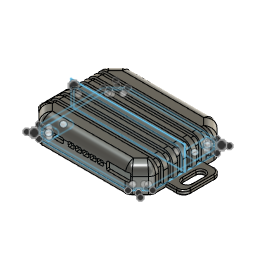
stm32-sensorleap-box-v12 (Autodesk Fusion 360 design; units mm, degrees)
Autodesk Fusion 360 part; units mm, degrees
sketch "Sketch1" plane through (0, 0, 0) normal (0, 0, 1) x (1, 0, 0) in component "lid"
  line L0 (-17.6716, 17.5) -> (17.6716, 17.5)
  line L1 (22, 13.1716) -> (22, -13.1716)
  line L2 (17.6716, -17.5) -> (-17.6716, -17.5)
  line L3 (-22, -13.1716) -> (-22, 13.1716)
  line L4 (-17.5574, 18.8) -> (17.5574, 18.8)
  line L5 (24, 12.3574) -> (24, -12.3074)
  line L6 (17.5574, -18.75) -> (-17.5574, -18.75)
  line L7 (-24, -12.3074) -> (-24, 12.3574)
  line L8 (19.0858, 16.9142) -> (21.4142, 14.5858)
  line L9 (21.4142, -14.5858) -> (19.0858, -16.9142)
  line L10 (-19.0858, -16.9142) -> (-21.4142, -14.5858)
  line L11 (-19.0858, 16.9142) -> (-21.4142, 14.5858)
  line L12 (19.6787, 17.9213) -> (23.1213, 14.4787)
  line L13 (23.1213, -14.4287) -> (19.6787, -17.8713)
  line L14 (-19.6787, -17.8713) -> (-23.1213, -14.4287)
  line L15 (-19.6787, 17.9213) -> (-23.1213, 14.4787)
  arc A0 (19.0858, 16.9142) -> (17.6716, 17.5) centre (17.6716, 15.5) ccw
  arc A1 (22, 13.1716) -> (21.4142, 14.5858) centre (20, 13.1716) ccw
  arc A2 (21.4142, -14.5858) -> (22, -13.1716) centre (20, -13.1716) ccw
  arc A3 (17.6716, -17.5) -> (19.0858, -16.9142) centre (17.6716, -15.5) ccw
  arc A4 (-19.0858, -16.9142) -> (-17.6716, -17.5) centre (-17.6716, -15.5) ccw
  arc A5 (-22, -13.1716) -> (-21.4142, -14.5858) centre (-20, -13.1716) ccw
  arc A6 (-21.4142, 14.5858) -> (-22, 13.1716) centre (-20, 13.1716) ccw
  arc A7 (-17.6716, 17.5) -> (-19.0858, 16.9142) centre (-17.6716, 15.5) ccw
  arc A8 (19.6787, 17.9213) -> (17.5574, 18.8) centre (17.5574, 15.8) ccw
  arc A9 (24, 12.3574) -> (23.1213, 14.4787) centre (21, 12.3574) ccw
  arc A10 (23.1213, -14.4287) -> (24, -12.3074) centre (21, -12.3074) ccw
  arc A11 (17.5574, -18.75) -> (19.6787, -17.8713) centre (17.5574, -15.75) ccw
  arc A12 (-19.6787, -17.8713) -> (-17.5574, -18.75) centre (-17.5574, -15.75) ccw
  arc A13 (-24, -12.3074) -> (-23.1213, -14.4287) centre (-21, -12.3074) ccw
  arc A14 (-23.1213, 14.4787) -> (-24, 12.3574) centre (-21, 12.3574) ccw
  arc A15 (-17.5574, 18.8) -> (-19.6787, 17.9213) centre (-17.5574, 15.8) ccw
  point P0 (-22, 17.5)
  point P1 (22, 17.5)
  point P2 (22, -17.5)
  point P3 (-22, -17.5)
  point P4 (-24, 18.8)
  point P5 (24, 18.8)
  point P6 (24, -18.75)
  point P7 (-24, -18.75)
  point P8 (18.5, 17.5)
  point P9 (22, 14)
  point P10 (22, -14)
  point P11 (18.5, -17.5)
  point P12 (-18.5, -17.5)
  point P13 (-22, -14)
  point P14 (-18.5, 17.5)
  point P15 (-22, 14)
  point P16 (18.8, 18.8)
  point P17 (24, 13.6)
  point P18 (24, -13.55)
  point P19 (18.8, -18.75)
  point P20 (-18.8, -18.75)
  point P21 (-24, -13.55)
  point P22 (-18.8, 18.8)
  point P23 (-24, 13.6)
  dimension "d1" = 44
  dimension "d2" = 35
  dimension "d3" = 3.5
  dimension "d4" = 3.5
  dimension "d5" = 3.5
  dimension "d6" = 3.5
  dimension "d7" = 3.5
  dimension "d8" = 3.5
  dimension "d9" = 3.5
  dimension "d10" = 3.5
  dimension "d11" = 5.2
  dimension "d12" = 5.2
  dimension "d13" = 5.2
  dimension "d14" = 5.2
  dimension "d15" = 5.2
  dimension "d16" = 5.2
  dimension "d17" = 5.2
  dimension "d18" = 5.2
  dimension "d19" = 2
  dimension "d20" = 3
  constraint horizontal L0
  constraint vertical L1
  constraint horizontal L2
  constraint vertical L3
  constraint horizontal L4
  constraint vertical L5
  constraint horizontal L6
  constraint vertical L7
  constraint coincident P1 L0
  constraint coincident P1 L1
  constraint coincident P2 L1
  constraint coincident P2 L2
  constraint coincident P3 L2
  constraint coincident P3 L3
  constraint coincident P0 L0
  constraint coincident P0 L3
  constraint coincident P5 L4
  constraint coincident P5 L5
  constraint coincident P6 L5
  constraint coincident P6 L6
  constraint coincident P7 L6
  constraint coincident P7 L7
  constraint coincident P4 L4
  constraint coincident P4 L7
  constraint coincident L0 P8
  constraint coincident P8 L8
  constraint tangent L0 A0
  constraint tangent L8 A0
  constraint coincident P9 L8
  constraint coincident L1 P9
  constraint tangent L8 A1
  constraint tangent L1 A1
  constraint equal A0 A1
  constraint coincident L1 P10
  constraint coincident P10 L9
  constraint tangent L1 A2
  constraint tangent L9 A2
  constraint equal A0 A2
  constraint coincident P11 L9
  constraint coincident L2 P11
  constraint tangent L9 A3
  constraint tangent L2 A3
  constraint equal A0 A3
  constraint coincident L2 P12
  constraint coincident P12 L10
  constraint tangent L2 A4
  constraint tangent L10 A4
  constraint equal A0 A4
  constraint coincident P13 L10
  constraint coincident L3 P13
  constraint tangent L10 A5
  constraint tangent L3 A5
  constraint equal A0 A5
  constraint coincident L3 P15
  constraint coincident P15 L11
  constraint tangent L3 A6
  constraint tangent L11 A6
  constraint equal A0 A6
  constraint coincident P14 L11
  constraint coincident L0 P14
  constraint tangent L11 A7
  constraint tangent L0 A7
  constraint equal A0 A7
  constraint coincident L4 P16
  constraint coincident P16 L12
  constraint tangent L4 A8
  constraint tangent L12 A8
  constraint coincident P17 L12
  constraint coincident L5 P17
  constraint tangent L12 A9
  constraint tangent L5 A9
  constraint equal A8 A9
  constraint coincident L5 P18
  constraint coincident P18 L13
  constraint tangent L5 A10
  constraint tangent L13 A10
  constraint equal A8 A10
  constraint coincident P19 L13
  constraint coincident L6 P19
  constraint tangent L13 A11
  constraint tangent L6 A11
  constraint equal A8 A11
  constraint coincident L6 P20
  constraint coincident P20 L14
  constraint tangent L6 A12
  constraint tangent L14 A12
  constraint equal A8 A12
  constraint coincident P21 L14
  constraint coincident L7 P21
  constraint tangent L14 A13
  constraint tangent L7 A13
  constraint equal A8 A13
  constraint coincident L7 P23
  constraint coincident P23 L15
  constraint tangent L7 A14
  constraint tangent L15 A14
  constraint equal A8 A14
  constraint coincident P22 L15
  constraint coincident L4 P22
  constraint tangent L15 A15
  constraint tangent L4 A15
  constraint equal A8 A15
  measures "d1" distance of P0 P1
  measures "d2" distance of P0 P3
  measures "d3" distance of P1 P8
  measures "d4" distance of P1 P9
  measures "d5" distance of P2 P10
  measures "d6" distance of P2 P11
  measures "d7" distance of P3 P12
  measures "d8" distance of P3 P13
  measures "d9" distance of P0 P14
  measures "d10" distance of P0 P15
  measures "d11" distance of P5 P16
  measures "d12" distance of P5 P17
  measures "d13" distance of P6 P18
  measures "d14" distance of P6 P19
  measures "d15" distance of P7 P20
  measures "d16" distance of P7 P21
  measures "d17" distance of P4 P22
  measures "d18" distance of P4 P23
  measures "d19" radius of A0
  measures "d20" radius of A8
sketch "Sketch2" plane through (0, 0, 0) normal (0, 1, 0) x (1, 0, 0) in component "lid"
  line L0 (-24, -10) -> (24, -10)
  line L1 (24, -10) -> (24, 0)
  line L2 (24, 0) -> (-24, 0)
  line L3 (-24, 0) -> (-24, -10)
  line L4 (-22.8, 0) -> (22.8, 0)
  line L5 (22.8, 0) -> (22.8, -6)
  line L6 (20.8, -8) -> (-20.8, -8)
  line L7 (-22.8, -6) -> (-22.8, 0)
  arc A0 (20.8, -8) -> (22.8, -6) centre (20.8, -6) ccw
  arc A1 (-22.8, -6) -> (-20.8, -8) centre (-20.8, -6) ccw
  point P0 (-22.8, -8)
  dimension "d21" = 48
  dimension "d22" = 10
  dimension "d23" = 45.6
  dimension "d24" = 8
  dimension "d38" = 2
  constraint horizontal L0
  constraint vertical L1
  constraint horizontal L2
  constraint vertical L3
  constraint horizontal L4
  constraint vertical L5
  constraint horizontal L6
  constraint vertical L7
  constraint tangent L5 A0
  constraint tangent L6 A0
  constraint coincident P0 L6
  constraint coincident P0 L7
  constraint tangent L6 A1
  constraint tangent L7 A1
  constraint equal A0 A1
  measures "d21" distance of L0.start L0.end
  measures "d22" distance of L0.start L2.end
  measures "d23" distance of L4.start L4.end
  measures "d24" distance of L4.start P0
  measures "d38" radius of A0
sketch "Sketch3" plane through (0, 0, 0) normal (0, 0, 1) x (1, 0, 0) in component "lid"
  line L0 (19, 17.5) -> (16, 17.5)
  line L1 (16, 17.5) -> (16, 15.5)
  line L2 (19, 12.5) -> (22, 12.5)
  line L3 (22, 12.5) -> (22, 14.5)
  line L4 (-19, -17.5) -> (-16, -17.5)
  line L5 (-16, -17.5) -> (-16, -14.5)
  line L6 (-19, -11.5) -> (-22, -11.5)
  line L7 (-22, -11.5) -> (-22, -14.5)
  arc A0 (16, 15.5) -> (19, 12.5) centre (19, 15.5) ccw
  arc A1 (-16, -14.5) -> (-19, -11.5) centre (-19, -14.5) ccw
  circle A2 centre (19, 9.25) radius 1
  circle A3 centre (-19, -8.25) radius 1
  circle A4 centre (19, 14.4989) radius 1.25
  circle A5 centre (-19, -14.5102) radius 1.25
  line L8 (19, 17.5) -> (16, 17.5)
  line L9 (16, 17.5) -> (16, 9.25)
  line L10 (19, 6.25) -> (22, 6.25)
  line L11 (22, 6.25) -> (22, 14.5)
  line L12 (-19, -17.5) -> (-16, -17.5)
  line L13 (-16, -17.5) -> (-16, -8.25)
  line L14 (-19, -5.25) -> (-22, -5.25)
  line L15 (-22, -5.25) -> (-22, -14.5)
  arc A6 (16, 9.25) -> (19, 6.25) centre (19, 9.25) ccw
  arc A7 (-16, -8.25) -> (-19, -5.25) centre (-19, -8.25) ccw
  line L16 (-22, -14.5) -> (-19, -17.5)
  line L17 (-19, -17.5) -> (-22, -14.5)
  line L18 (19, 17.5) -> (22, 14.5)
  line L19 (19, 17.5) -> (22, 14.5)
  point P0 (22, 17.5)
  point P1 (-22, -17.5)
  dimension "d92" = 6
  dimension "d93" = 5
  dimension "d94" = 6
  dimension "d95" = 6
  dimension "d96" = 3
  dimension "d97" = 3
  dimension "d98" = 2
  dimension "d99" = 2
  dimension "d100" = 2.5
  dimension "d101" = 2.5
  dimension "d102" = 11.25
  dimension "d103" = 12.25
  dimension "d104" = 3
  dimension "d105" = 3
  dimension "d106" = 3
  dimension "d107" = 3
  dimension "d108" = 3
  dimension "d109" = 3
  dimension "d110" = 3
  dimension "d111" = 3
  dimension "d112" = 3
  dimension "d113" = 3
  constraint horizontal L0
  constraint vertical L1
  constraint horizontal L2
  constraint vertical L3
  constraint horizontal L4
  constraint vertical L5
  constraint horizontal L6
  constraint vertical L7
  constraint tangent L2 A0
  constraint tangent L1 A0
  constraint tangent L6 A1
  constraint tangent L5 A1
  constraint horizontal L8
  constraint vertical L9
  constraint horizontal L10
  constraint vertical L11
  constraint horizontal L12
  constraint vertical L13
  constraint horizontal L14
  constraint vertical L15
  constraint tangent L10 A6
  constraint tangent L9 A6
  constraint tangent L13 A7
  constraint tangent L14 A7
  constraint coincident P1 L15
  constraint coincident P1 L12
  constraint coincident P1 L4
  constraint coincident P1 L7
  constraint coincident P0 L0
  constraint coincident P0 L3
  constraint coincident P0 L8
  constraint coincident P0 L11
  measures "d92" distance of P0 L0.end
  measures "d93" distance of P0 L2.end
  measures "d94" distance of P1 L4.end
  measures "d95" distance of P1 L6.end
  measures "d96" radius of A0
  measures "d97" radius of A1
  measures "d98" diameter of A2
  measures "d99" diameter of A3
  measures "d100" diameter of A4
  measures "d101" diameter of A5
  measures "d102" distance of P0 L10.end
  measures "d103" distance of P1 L14.end
  measures "d104" radius of A6
  measures "d105" radius of A7
  measures "d106" distance of P1 L7.end
  measures "d107" distance of P1 L4.start
  measures "d108" distance of P1 L4.start
  measures "d109" distance of P1 L7.end
  measures "d110" distance of P0 L0.start
  measures "d111" distance of P0 L3.end
  measures "d112" distance of P0 L0.start
  measures "d113" distance of P0 L3.end
sketch "sma" plane through (0, 0, 0) normal (0, 1, 0) x (1, 0, 0) in component "lid"
  line L0 (-8.6, -6.9972) -> (-15.1, -6.9972)
  line L1 (-15.1, -6.9972) -> (-15.1, 1.5028)
  line L2 (-15.1, 1.5028) -> (-8.6, 1.5028)
  line L3 (-8.6, 1.5028) -> (-8.6, -6.9972)
  dimension "d121" = 8.5
  constraint horizontal L0
  constraint vertical L1
  constraint horizontal L2
  constraint vertical L3
  measures "d121" distance of L0.start L2.end
sketch "panel" plane through (0, 0, 0) normal (0, 1, 0) x (1, 0, 0) in component "lid"
  line L0 (10.2, -6.2) -> (18.8, -6.2)
  line L1 (19.3, -5.7) -> (19.3, -3.3)
  line L2 (18.8, -2.8) -> (10.2, -2.8)
  line L3 (9.7, -3.3) -> (9.7, -5.7)
  line L4 (4.8, -5.4) -> (3.3, -5.4)
  line L5 (2.8, -4.9) -> (2.8, -3.9)
  line L6 (3.3, -3.4) -> (4.8, -3.4)
  line L7 (5.3, -3.9) -> (5.3, -4.9)
  line L8 (1.7, -5.4) -> (0.2, -5.4)
  line L9 (-0.3, -4.9) -> (-0.3, -3.9)
  line L10 (0.2, -3.4) -> (1.7, -3.4)
  line L11 (2.2, -3.9) -> (2.2, -4.9)
  line L12 (-1.4, -5.4) -> (-2.9, -5.4)
  line L13 (-3.4, -4.9) -> (-3.4, -3.9)
  line L14 (-2.9, -3.4) -> (-1.4, -3.4)
  line L15 (-0.9, -3.9) -> (-0.9, -4.9)
  line L16 (-4.5, -5.4) -> (-6, -5.4)
  line L17 (-6.5, -4.9) -> (-6.5, -3.9)
  line L18 (-6, -3.4) -> (-4.5, -3.4)
  line L19 (-4, -3.9) -> (-4, -4.9)
  line L20 (-9, -5.3) -> (-12.5, -5.3)
  line L21 (-13, -4.8) -> (-13, -3.7)
  line L22 (-12.5, -3.2) -> (-9, -3.2)
  line L23 (-8.5, -3.7) -> (-8.5, -4.8)
  arc A0 (18.8, -6.2) -> (19.3, -5.7) centre (18.8, -5.7) ccw
  arc A1 (19.3, -3.3) -> (18.8, -2.8) centre (18.8, -3.3) ccw
  arc A2 (10.2, -2.8) -> (9.7, -3.3) centre (10.2, -3.3) ccw
  arc A3 (9.7, -5.7) -> (10.2, -6.2) centre (10.2, -5.7) ccw
  arc A4 (4.8, -5.4) -> (5.3, -4.9) centre (4.8, -4.9) ccw
  arc A5 (5.3, -3.9) -> (4.8, -3.4) centre (4.8, -3.9) ccw
  arc A6 (3.3, -3.4) -> (2.8, -3.9) centre (3.3, -3.9) ccw
  arc A7 (2.8, -4.9) -> (3.3, -5.4) centre (3.3, -4.9) ccw
  arc A8 (1.7, -5.4) -> (2.2, -4.9) centre (1.7, -4.9) ccw
  arc A9 (2.2, -3.9) -> (1.7, -3.4) centre (1.7, -3.9) ccw
  arc A10 (0.2, -3.4) -> (-0.3, -3.9) centre (0.2, -3.9) ccw
  arc A11 (-0.3, -4.9) -> (0.2, -5.4) centre (0.2, -4.9) ccw
  arc A12 (-1.4, -5.4) -> (-0.9, -4.9) centre (-1.4, -4.9) ccw
  arc A13 (-0.9, -3.9) -> (-1.4, -3.4) centre (-1.4, -3.9) ccw
  arc A14 (-2.9, -3.4) -> (-3.4, -3.9) centre (-2.9, -3.9) ccw
  arc A15 (-3.4, -4.9) -> (-2.9, -5.4) centre (-2.9, -4.9) ccw
  arc A16 (-4.5, -5.4) -> (-4, -4.9) centre (-4.5, -4.9) ccw
  arc A17 (-4, -3.9) -> (-4.5, -3.4) centre (-4.5, -3.9) ccw
  arc A18 (-6, -3.4) -> (-6.5, -3.9) centre (-6, -3.9) ccw
  arc A19 (-6.5, -4.9) -> (-6, -5.4) centre (-6, -4.9) ccw
  arc A20 (-9, -5.3) -> (-8.5, -4.8) centre (-9, -4.8) ccw
  arc A21 (-8.5, -3.7) -> (-9, -3.2) centre (-9, -3.7) ccw
  arc A22 (-12.5, -3.2) -> (-13, -3.7) centre (-12.5, -3.7) ccw
  arc A23 (-13, -4.8) -> (-12.5, -5.3) centre (-12.5, -4.8) ccw
  line L24 (7.9, -3.4) -> (6.4, -3.4)
  line L25 (5.9, -3.9) -> (5.9, -4.9)
  line L26 (6.4, -5.4) -> (7.9, -5.4)
  line L27 (8.4, -4.9) -> (8.4, -3.9)
  arc A24 (6.4, -3.4) -> (5.9, -3.9) centre (6.4, -3.9) ccw
  arc A25 (5.9, -4.9) -> (6.4, -5.4) centre (6.4, -4.9) ccw
  arc A26 (7.9, -5.4) -> (8.4, -4.9) centre (7.9, -4.9) ccw
  arc A27 (8.4, -3.9) -> (7.9, -3.4) centre (7.9, -3.9) ccw
  point P0 (9.7, -6.2)
  point P1 (19.3, -6.2)
  point P2 (9.7, -2.8)
  point P3 (5.3, -5.4)
  point P4 (2.8, -5.4)
  point P5 (2.2, -5.4)
  point P6 (-0.3, -5.4)
  point P7 (2.2, -3.4)
  point P8 (-0.9, -5.4)
  point P9 (-3.4, -5.4)
  point P10 (-4, -5.4)
  point P11 (-6.5, -5.4)
  point P12 (-4, -3.4)
  point P13 (-8.5, -5.3)
  point P14 (-13, -5.3)
  point P15 (-8.5, -3.2)
  point P16 (8.4, -3.4)
  point P17 (5.9, -3.4)
  point P18 (8.4, -5.4)
  dimension "d125" = 9.6
  dimension "d126" = 3.4
  dimension "d127" = 2.5
  dimension "d128" = 2.5
  dimension "d129" = 2
  dimension "d130" = 2.5
  dimension "d131" = 2.5
  dimension "d132" = 2
  dimension "d133" = 4.5
  dimension "d134" = 2.1
  dimension "d138" = 0.5
  dimension "d139" = 2.5
  dimension "d140" = 2
  dimension "d141" = 0.5
  constraint horizontal L0
  constraint vertical L1
  constraint horizontal L2
  constraint vertical L3
  constraint horizontal L4
  constraint vertical L5
  constraint horizontal L6
  constraint vertical L7
  constraint horizontal L8
  constraint vertical L9
  constraint horizontal L10
  constraint vertical L11
  constraint horizontal L12
  constraint vertical L13
  constraint horizontal L14
  constraint vertical L15
  constraint horizontal L16
  constraint vertical L17
  constraint horizontal L18
  constraint vertical L19
  constraint horizontal L20
  constraint vertical L21
  constraint horizontal L22
  constraint vertical L23
  constraint coincident P1 L0
  constraint coincident P1 L1
  constraint tangent L0 A0
  constraint tangent L1 A0
  constraint tangent L1 A1
  constraint tangent L2 A1
  constraint equal A0 A1
  constraint coincident P2 L2
  constraint coincident P2 L3
  constraint tangent L2 A2
  constraint tangent L3 A2
  constraint equal A0 A2
  constraint coincident P0 L3
  constraint coincident P0 L0
  constraint tangent L3 A3
  constraint tangent L0 A3
  constraint equal A0 A3
  constraint coincident P3 L4
  constraint coincident P3 L7
  constraint tangent L4 A4
  constraint tangent L7 A4
  constraint equal A0 A4
  constraint tangent L7 A5
  constraint tangent L6 A5
  constraint equal A0 A5
  constraint tangent L6 A6
  constraint tangent L5 A6
  constraint equal A0 A6
  constraint coincident P4 L5
  constraint coincident P4 L4
  constraint tangent L5 A7
  constraint tangent L4 A7
  constraint equal A0 A7
  constraint coincident P5 L8
  constraint coincident P5 L11
  constraint tangent L8 A8
  constraint tangent L11 A8
  constraint equal A0 A8
  constraint coincident P7 L11
  constraint coincident P7 L10
  constraint tangent L11 A9
  constraint tangent L10 A9
  constraint equal A0 A9
  constraint tangent L10 A10
  constraint tangent L9 A10
  constraint equal A0 A10
  constraint coincident P6 L9
  constraint coincident P6 L8
  constraint tangent L9 A11
  constraint tangent L8 A11
  constraint equal A0 A11
  constraint coincident P8 L12
  constraint coincident P8 L15
  constraint tangent L12 A12
  constraint tangent L15 A12
  constraint equal A0 A12
  constraint tangent L15 A13
  constraint tangent L14 A13
  constraint equal A0 A13
  constraint tangent L14 A14
  constraint tangent L13 A14
  constraint equal A0 A14
  constraint coincident P9 L13
  constraint coincident P9 L12
  constraint tangent L13 A15
  constraint tangent L12 A15
  constraint equal A0 A15
  constraint coincident P10 L16
  constraint coincident P10 L19
  constraint tangent L16 A16
  constraint tangent L19 A16
  constraint equal A0 A16
  constraint coincident P12 L19
  constraint coincident P12 L18
  constraint tangent L19 A17
  constraint tangent L18 A17
  constraint equal A0 A17
  constraint tangent L18 A18
  constraint tangent L17 A18
  constraint equal A0 A18
  constraint coincident P11 L17
  constraint coincident P11 L16
  constraint tangent L17 A19
  constraint tangent L16 A19
  constraint equal A0 A19
  constraint coincident P13 L20
  constraint coincident P13 L23
  constraint tangent L20 A20
  constraint tangent L23 A20
  constraint equal A0 A20
  constraint coincident P15 L23
  constraint coincident P15 L22
  constraint tangent L23 A21
  constraint tangent L22 A21
  constraint equal A0 A21
  constraint tangent L22 A22
  constraint tangent L21 A22
  constraint equal A0 A22
  constraint coincident P14 L21
  constraint coincident P14 L20
  constraint tangent L21 A23
  constraint tangent L20 A23
  constraint equal A0 A23
  constraint horizontal L24
  constraint vertical L25
  constraint horizontal L26
  constraint vertical L27
  constraint coincident P17 L25
  constraint coincident P17 L24
  constraint tangent L25 A24
  constraint tangent L24 A24
  constraint tangent L25 A25
  constraint tangent L26 A25
  constraint equal A24 A25
  constraint coincident P18 L26
  constraint coincident P18 L27
  constraint tangent L26 A26
  constraint tangent L27 A26
  constraint equal A24 A26
  constraint coincident P16 L27
  constraint coincident P16 L24
  constraint tangent L27 A27
  constraint tangent L24 A27
  constraint equal A24 A27
  measures "d125" distance of P0 P1
  measures "d126" distance of P0 P2
  measures "d127" distance of P3 P4
  measures "d128" distance of P5 P6
  measures "d129" distance of P5 P7
  measures "d130" distance of P8 P9
  measures "d131" distance of P10 P11
  measures "d132" distance of P10 P12
  measures "d133" distance of P13 P14
  measures "d134" distance of P13 P15
  measures "d138" radius of A0
  measures "d139" distance of P16 P17
  measures "d140" distance of P16 P18
  measures "d141" radius of A24
extrude "Extrude1" add sketch "Sketch1" along normal blind 9 makes body 1 in component "lid"
extrude "Extrude2" add sketch "Sketch1" along normal blind 2 from surface at 7 contours L0 L1 L2 L3 L8 L9 L10 L11 A0 A1 A2 A3 A4 A5 A6 A7 | L4 L5 L6 L7 L12 L13 L14 L15 A8 A9 A10 A11 A12 A13 A14 A15 bodies 1 in component "lid"
fillet "Fillet1" radius 4 16 edges at (21.4, -16.15, 9) (23.7716, -13.4554, 9) (24, 0.025, 9) (23.7716, 13.5054, 9) (21.4, 16.2, 9) (18.7054, 18.5716, 9) (0, 18.8, 9) (-18.7054, 18.5716, 9) (-21.4, 16.2, 9) (-23.7716, 13.5054, 9) (-24, 0.025, 9) (-23.7716, -13.4554, 9) (-21.4, -16.15, 9) (-18.7054, -18.5216, 9) (0, -18.75, 9) (18.7054, -18.5216, 9) on bodies 1 in component "lid"
extrude "Extrude3" add sketch "Sketch2" along normal blind 2 separate body contours L0 L1 L2 L3 L5 L6 L7 A0 A1 makes body 2 in component "lid"
pattern_linear "R-Pattern1" count 6 spacing 4 along (0, 1, 0) of bodies 2 makes body 3 at (-6.9333, 4, 9.3333) makes body 4 at (-6.9333, 8, 9.3333) makes body 5 at (-6.9333, 12, 9.3333) makes body 6 at (-6.9333, 16, 9.3333) makes body 7 at (-6.9333, 20, 9.3333) in component "lid"
move_body "Move1" bodies 3 4 7 2 5 6 to x (1, 0, 0) y (0, 1, 0) z (0, 0, 1) at (0, -11, 0) in component "lid"
combine "Combine1" operation cut target body 1 tool bodies 2 3 4 5 6 7 in component "lid"
sketch "Sketch1 (2)" plane through (0, 0, 0) normal (0, 0, 1) x (1, 0, 0) in component "base"
  line L0 (-17.5574, 18.75) -> (17.5574, 18.75)
  line L1 (24, 12.3074) -> (24, -12.3074)
  line L2 (17.5574, -18.75) -> (-17.5574, -18.75)
  line L3 (-24, -12.3074) -> (-24, 12.3074)
  line L4 (19.6787, 17.8713) -> (23.1213, 14.4287)
  line L5 (23.1213, -14.4287) -> (19.6787, -17.8713)
  line L6 (-19.6787, -17.8713) -> (-23.1213, -14.4287)
  line L7 (-19.6787, 17.8713) -> (-23.1213, 14.4287)
  arc A0 (19.6787, 17.8713) -> (17.5574, 18.75) centre (17.5574, 15.75) ccw
  arc A1 (24, 12.3074) -> (23.1213, 14.4287) centre (21, 12.3074) ccw
  arc A2 (23.1213, -14.4287) -> (24, -12.3074) centre (21, -12.3074) ccw
  arc A3 (17.5574, -18.75) -> (19.6787, -17.8713) centre (17.5574, -15.75) ccw
  arc A4 (-19.6787, -17.8713) -> (-17.5574, -18.75) centre (-17.5574, -15.75) ccw
  arc A5 (-24, -12.3074) -> (-23.1213, -14.4287) centre (-21, -12.3074) ccw
  arc A6 (-23.1213, 14.4287) -> (-24, 12.3074) centre (-21, 12.3074) ccw
  arc A7 (-17.5574, 18.75) -> (-19.6787, 17.8713) centre (-17.5574, 15.75) ccw
  line L8 (24, 8) -> (28.5, 8)
  line L9 (31.5, 5) -> (31.5, -5)
  line L10 (28.5, -8) -> (24, -8)
  line L11 (24, -8) -> (24, 8)
  arc A8 (31.5, 5) -> (28.5, 8) centre (28.5, 5) ccw
  arc A9 (28.5, -8) -> (31.5, -5) centre (28.5, -5) ccw
  line L12 (-24, 8) -> (-28.5, 8)
  line L13 (-31.5, 5) -> (-31.5, -5)
  line L14 (-28.5, -8) -> (-24, -8)
  line L15 (-24, -8) -> (-24, 8)
  arc A10 (-28.5, 8) -> (-31.5, 5) centre (-28.5, 5) ccw
  arc A11 (-31.5, -5) -> (-28.5, -8) centre (-28.5, -5) ccw
  line L16 (-17.6716, 17.5) -> (17.6716, 17.5)
  line L17 (22, 13.1716) -> (22, -13.1716)
  line L18 (17.6716, -17.5) -> (-17.6716, -17.5)
  line L19 (-22, -13.1716) -> (-22, 13.1716)
  line L20 (-18.0858, 17) -> (18.0858, 17)
  line L21 (21.5, 13.5858) -> (21.5, -13.5858)
  line L22 (18.0858, -17) -> (-18.0858, -17)
  line L23 (-21.5, -13.5858) -> (-21.5, 13.5858)
  line L24 (-19.0858, 16.9142) -> (-21.4142, 14.5858)
  line L25 (19.0858, 16.9142) -> (21.4142, 14.5858)
  line L26 (21.4142, -14.5858) -> (19.0858, -16.9142)
  line L27 (-19.0858, -16.9142) -> (-21.4142, -14.5858)
  line L28 (18.7929, 16.7071) -> (21.2071, 14.2929)
  line L29 (21.2071, -14.2929) -> (18.7929, -16.7071)
  line L30 (-18.7929, -16.7071) -> (-21.2071, -14.2929)
  line L31 (-18.7929, 16.7071) -> (-21.2071, 14.2929)
  arc A12 (19.0858, 16.9142) -> (17.6716, 17.5) centre (17.6716, 15.5) ccw
  arc A13 (22, 13.1716) -> (21.4142, 14.5858) centre (20, 13.1716) ccw
  arc A14 (21.4142, -14.5858) -> (22, -13.1716) centre (20, -13.1716) ccw
  arc A15 (17.6716, -17.5) -> (19.0858, -16.9142) centre (17.6716, -15.5) ccw
  arc A16 (-19.0858, -16.9142) -> (-17.6716, -17.5) centre (-17.6716, -15.5) ccw
  arc A17 (-22, -13.1716) -> (-21.4142, -14.5858) centre (-20, -13.1716) ccw
  arc A18 (-21.4142, 14.5858) -> (-22, 13.1716) centre (-20, 13.1716) ccw
  arc A19 (-17.6716, 17.5) -> (-19.0858, 16.9142) centre (-17.6716, 15.5) ccw
  arc A20 (18.7929, 16.7071) -> (18.0858, 17) centre (18.0858, 16) ccw
  arc A21 (21.5, 13.5858) -> (21.2071, 14.2929) centre (20.5, 13.5858) ccw
  arc A22 (21.2071, -14.2929) -> (21.5, -13.5858) centre (20.5, -13.5858) ccw
  arc A23 (18.0858, -17) -> (18.7929, -16.7071) centre (18.0858, -16) ccw
  arc A24 (-18.7929, -16.7071) -> (-18.0858, -17) centre (-18.0858, -16) ccw
  arc A25 (-21.5, -13.5858) -> (-21.2071, -14.2929) centre (-20.5, -13.5858) ccw
  arc A26 (-21.2071, 14.2929) -> (-21.5, 13.5858) centre (-20.5, 13.5858) ccw
  arc A27 (-18.0858, 17) -> (-18.7929, 16.7071) centre (-18.0858, 16) ccw
  line L32 (29.5, 2.75) -> (29.5, -2.75)
  line L33 (26, -2.75) -> (26, 2.75)
  line L34 (-29.5, 2.75) -> (-29.5, -2.75)
  line L35 (-26, -2.75) -> (-26, 2.75)
  arc A28 (-26, 2.75) -> (-27.75, 4.5) centre (-27.75, 2.75) ccw
  arc A29 (-27.75, -4.5) -> (-26, -2.75) centre (-27.75, -2.75) ccw
  arc A30 (-29.5, -2.75) -> (-27.75, -4.5) centre (-27.75, -2.75) ccw
  arc A31 (-27.75, 4.5) -> (-29.5, 2.75) centre (-27.75, 2.75) ccw
  arc A32 (29.5, 2.75) -> (27.75, 4.5) centre (27.75, 2.75) ccw
  arc A33 (27.75, -4.5) -> (29.5, -2.75) centre (27.75, -2.75) ccw
  arc A34 (26, -2.75) -> (27.75, -4.5) centre (27.75, -2.75) ccw
  arc A35 (27.75, 4.5) -> (26, 2.75) centre (27.75, 2.75) ccw
  point P0 (-24, 18.75)
  point P1 (24, 18.75)
  point P2 (24, -18.75)
  point P3 (-24, -18.75)
  point P4 (18.8, 18.75)
  point P5 (24, 13.55)
  point P6 (24, -13.55)
  point P7 (18.8, -18.75)
  point P8 (-18.8, -18.75)
  point P9 (-24, -13.55)
  point P10 (-18.8, 18.75)
  point P11 (-24, 13.55)
  point P12 (31.5, 8)
  point P13 (-31.5, 8)
  point P14 (-22, 17.5)
  point P15 (22, 17.5)
  point P16 (22, -17.5)
  point P17 (-22, -17.5)
  point P18 (-21.5, 17)
  point P19 (21.5, 17)
  point P20 (21.5, -17)
  point P21 (-21.5, -17)
  point P22 (-18.5, 17.5)
  point P23 (-22, 14)
  point P24 (18.5, 17.5)
  point P25 (22, 14)
  point P26 (22, -14)
  point P27 (18.5, -17.5)
  point P28 (-18.5, -17.5)
  point P29 (-22, -14)
  point P30 (18.5, 17)
  point P31 (21.5, 14)
  point P32 (21.5, -14)
  point P33 (18.5, -17)
  point P34 (-18.5, -17)
  point P35 (-21.5, -14)
  point P36 (-18.5, 17)
  point P37 (-21.5, 14)
  point P38 (26, 4.5)
  point P39 (29.5, 4.5)
  point P40 (26, -4.5)
  point P41 (-26, 4.5)
  point P42 (-29.5, 4.5)
  point P43 (-26, -4.5)
  dimension "d39" = 5.2
  dimension "d40" = 5.2
  dimension "d41" = 5.2
  dimension "d42" = 5.2
  dimension "d43" = 5.2
  dimension "d44" = 5.2
  dimension "d45" = 5.2
  dimension "d46" = 5.2
  dimension "d47" = 3
  dimension "d48" = 7.5
  dimension "d49" = 16
  dimension "d50" = 3
  dimension "d51" = 7.5
  dimension "d52" = 16
  dimension "d53" = 3
  dimension "d54" = 3.5
  dimension "d55" = 3.5
  dimension "d56" = 3.5
  dimension "d57" = 3.5
  dimension "d58" = 3.5
  dimension "d59" = 3.5
  dimension "d60" = 3.5
  dimension "d61" = 3.5
  dimension "d62" = 3
  dimension "d63" = 3
  dimension "d64" = 3
  dimension "d65" = 3
  dimension "d66" = 3
  dimension "d67" = 3
  dimension "d68" = 3
  dimension "d69" = 3
  dimension "d70" = 2
  dimension "d71" = 1
  dimension "d72" = 3.5
  dimension "d73" = 9
  dimension "d74" = 3.5
  dimension "d75" = 9
  dimension "d76" = 1.75
  dimension "d77" = 1.75
  constraint horizontal L0
  constraint vertical L1
  constraint horizontal L2
  constraint vertical L3
  constraint coincident P1 L0
  constraint coincident P1 L1
  constraint coincident P2 L1
  constraint coincident P2 L2
  constraint coincident P3 L2
  constraint coincident P3 L3
  constraint coincident P0 L0
  constraint coincident P0 L3
  constraint coincident L0 P4
  constraint coincident P4 L4
  constraint tangent L0 A0
  constraint tangent L4 A0
  constraint coincident P5 L4
  constraint coincident L1 P5
  constraint tangent L4 A1
  constraint tangent L1 A1
  constraint equal A0 A1
  constraint coincident L1 P6
  constraint coincident P6 L5
  constraint tangent L1 A2
  constraint tangent L5 A2
  constraint equal A0 A2
  constraint coincident P7 L5
  constraint coincident L2 P7
  constraint tangent L5 A3
  constraint tangent L2 A3
  constraint equal A0 A3
  constraint coincident L2 P8
  constraint coincident P8 L6
  constraint tangent L2 A4
  constraint tangent L6 A4
  constraint equal A0 A4
  constraint coincident P9 L6
  constraint coincident L3 P9
  constraint tangent L6 A5
  constraint tangent L3 A5
  constraint equal A0 A5
  constraint coincident L3 P11
  constraint coincident P11 L7
  constraint tangent L3 A6
  constraint tangent L7 A6
  constraint equal A0 A6
  constraint coincident P10 L7
  constraint coincident L0 P10
  constraint tangent L7 A7
  constraint tangent L0 A7
  constraint equal A0 A7
  constraint horizontal L8
  constraint vertical L9
  constraint horizontal L10
  constraint vertical L11
  constraint coincident L1 L8.start
  constraint coincident P12 L8
  constraint coincident P12 L9
  constraint tangent L8 A8
  constraint tangent L9 A8
  constraint tangent L9 A9
  constraint tangent L10 A9
  constraint equal A8 A9
  constraint horizontal L12
  constraint vertical L13
  constraint horizontal L14
  constraint vertical L15
  constraint coincident L3 L12.start
  constraint coincident P13 L12
  constraint coincident P13 L13
  constraint tangent L12 A10
  constraint tangent L13 A10
  constraint tangent L13 A11
  constraint tangent L14 A11
  constraint equal A10 A11
  constraint horizontal L16
  constraint vertical L17
  constraint horizontal L18
  constraint vertical L19
  constraint horizontal L20
  constraint vertical L21
  constraint horizontal L22
  constraint vertical L23
  constraint coincident P14 L16
  constraint coincident P14 L19
  constraint coincident P15 L16
  constraint coincident P15 L17
  constraint coincident P16 L17
  constraint coincident P16 L18
  constraint coincident P17 L18
  constraint coincident P17 L19
  constraint coincident P19 L20
  constraint coincident P19 L21
  constraint coincident P20 L21
  constraint coincident P20 L22
  constraint coincident P21 L22
  constraint coincident P21 L23
  constraint coincident P18 L20
  constraint coincident P18 L23
  constraint coincident L16 P24
  constraint coincident P24 L25
  constraint tangent L16 A12
  constraint tangent L25 A12
  constraint coincident P25 L25
  constraint coincident L17 P25
  constraint tangent L25 A13
  constraint tangent L17 A13
  constraint equal A12 A13
  constraint coincident L17 P26
  constraint coincident P26 L26
  constraint tangent L17 A14
  constraint tangent L26 A14
  constraint equal A12 A14
  constraint coincident P27 L26
  constraint coincident L18 P27
  constraint tangent L26 A15
  constraint tangent L18 A15
  constraint equal A12 A15
  constraint coincident L18 P28
  constraint coincident P28 L27
  constraint tangent L18 A16
  constraint tangent L27 A16
  constraint equal A12 A16
  constraint coincident P29 L27
  constraint coincident L19 P29
  constraint tangent L27 A17
  constraint tangent L19 A17
  constraint equal A12 A17
  constraint coincident L19 P23
  constraint coincident P23 L24
  constraint tangent L19 A18
  constraint tangent L24 A18
  constraint equal A12 A18
  constraint coincident P22 L24
  constraint coincident L16 P22
  constraint tangent L24 A19
  constraint tangent L16 A19
  constraint equal A12 A19
  constraint coincident L20 P30
  constraint coincident P30 L28
  constraint tangent L20 A20
  constraint tangent L28 A20
  constraint coincident P31 L28
  constraint coincident L21 P31
  constraint tangent L28 A21
  constraint tangent L21 A21
  constraint equal A20 A21
  constraint coincident L21 P32
  constraint coincident P32 L29
  constraint tangent L21 A22
  constraint tangent L29 A22
  constraint equal A20 A22
  constraint coincident P33 L29
  constraint coincident L22 P33
  constraint tangent L29 A23
  constraint tangent L22 A23
  constraint equal A20 A23
  constraint coincident L22 P34
  constraint coincident P34 L30
  constraint tangent L22 A24
  constraint tangent L30 A24
  constraint equal A20 A24
  constraint coincident P35 L30
  constraint coincident L23 P35
  constraint tangent L30 A25
  constraint tangent L23 A25
  constraint equal A20 A25
  constraint coincident L23 P37
  constraint coincident P37 L31
  constraint tangent L23 A26
  constraint tangent L31 A26
  constraint equal A20 A26
  constraint coincident P36 L31
  constraint coincident L20 P36
  constraint tangent L31 A27
  constraint tangent L20 A27
  constraint equal A20 A27
  constraint vertical L32
  constraint vertical L33
  constraint vertical L34
  constraint vertical L35
  constraint coincident P41 L35
  constraint tangent L35 A28
  constraint coincident P43 L35
  constraint tangent L35 A29
  constraint equal A28 A29
  constraint tangent L34 A30
  constraint equal A28 A30
  constraint coincident A29.start A30.end
  constraint coincident P42 L34
  constraint tangent L34 A31
  constraint equal A28 A31
  constraint coincident A28.end A31.start
  constraint coincident P39 L32
  constraint tangent L32 A32
  constraint tangent L32 A33
  constraint equal A32 A33
  constraint coincident P40 L33
  constraint tangent L33 A34
  constraint equal A32 A34
  constraint coincident A33.start A34.end
  constraint coincident P38 L33
  constraint tangent L33 A35
  constraint equal A32 A35
  constraint coincident A32.end A35.start
  measures "d39" distance of P1 P4
  measures "d40" distance of P1 P5
  measures "d41" distance of P2 P6
  measures "d42" distance of P2 P7
  measures "d43" distance of P3 P8
  measures "d44" distance of P3 P9
  measures "d45" distance of P0 P10
  measures "d46" distance of P0 P11
  measures "d47" radius of A0
  measures "d48" distance of L8.start P12
  measures "d49" distance of L8.start L10.end
  measures "d50" radius of A8
  measures "d51" distance of L12.start P13
  measures "d52" distance of L12.start L14.end
  measures "d53" radius of A10
  measures "d54" distance of P14 P22
  measures "d55" distance of P14 P23
  measures "d56" distance of P15 P24
  measures "d57" distance of P15 P25
  measures "d58" distance of P16 P26
  measures "d59" distance of P16 P27
  measures "d60" distance of P17 P28
  measures "d61" distance of P17 P29
  measures "d62" distance of P19 P30
  measures "d63" distance of P19 P31
  measures "d64" distance of P20 P32
  measures "d65" distance of P20 P33
  measures "d66" distance of P21 P34
  measures "d67" distance of P21 P35
  measures "d68" distance of P18 P36
  measures "d69" distance of P18 P37
  measures "d70" radius of A12
  measures "d71" radius of A20
  measures "d72" distance of P38 P39
  measures "d73" distance of P38 P40
  measures "d74" distance of P41 P42
  measures "d75" distance of P41 P43
  measures "d76" radius of A28
  measures "d77" radius of A32
extrude "Extrude1'" add sketch "Sketch1 (2)" against normal blind 2 separate body contours L0 L1 L2 L3 L4 L5 L6 L7 A0 A1 A2 A3 A4 A5 A6 A7 L11 L15 | L3 L12 L13 L14 L15 A10 A11 | L1 L8 L9 L10 L11 A8 A9 | L16 L17 L18 L19 L24 L25 L26 L27 A12 A13 A14 A15 A16 A17 A18 A19 | L20 L21 L22 L23 L28 L29 L30 L31 A20 A21 A22 A23 A24 A25 A26 A27 | L32 L33 A32 A33 A34 A35 | L34 L35 A28 A29 A30 A31 makes body 8 in component "base"
extrude "Extrude2'" add sketch "Sketch1 (2)" along normal blind 1.5 contours L16 L17 L18 L19 L24 L25 L26 L27 A12 A13 A14 A15 A16 A17 A18 A19 bodies 8 in component "base"
extrude "Extrude3'" cut sketch "Sketch1 (2)" against normal blind 2 contours L32 L33 A32 A33 A34 A35 | L34 L35 A28 A29 A30 A31 bodies 8 in component "base"
fillet "Fillet1'" radius 0.5 19 edges at (24, -10.1537, -2) (23.7716, -13.4554, -2) (21.4, -16.15, -2) (18.7054, -18.5216, -2) (0, -18.75, -2) (-18.7054, -18.5216, -2) (-21.4, -16.15, -2) (-23.7716, -13.4554, -2) (-24, -10.1537, -2) (-26.25, -8, -2) (-30.6213, -7.1213, -2) (-31.5, 0, -2) (-30.6213, 7.1213, -2) (-26.25, 8, -2) (26.25, 8, -2) (30.6213, 7.1213, -2) (31.5, 0, -2) (30.6213, -7.1213, -2) (26.25, -8, -2) on bodies 8 in component "base"
fillet "Fillet2" radius 0.5 16 edges at (-29.5, 0, -2) (-27.75, -4.5, -2) (-26, 0, -2) (-27.75, 4.5, -2) (29.5, 0, -2) (27.75, 4.5, -2) (26, 0, -2) (27.75, -4.5, -2) (27.75, -4.5, 0) (26, 0, 0) (27.75, 4.5, 0) (29.5, 0, 0) (-27.75, -4.5, 0) (-29.5, 0, 0) (-27.75, 4.5, 0) (-26, 0, 0) on bodies 8 in component "base"
fillet "Fillet3" radius 0.5 10 edges at (-26.25, 8, 0) (-30.6213, 7.1213, 0) (-31.5, 0, 0) (-30.6213, -7.1213, 0) (-26.25, -8, 0) (26.25, 8, 0) (30.6213, 7.1213, 0) (31.5, 0, 0) (30.6213, -7.1213, 0) (26.25, -8, 0) on bodies 8 in component "base"
fillet "Fillet2'" radius 1 16 edges at (-20.25, 15.75, 7) (-21.8478, 13.9369, 7) (-22, 0, 7) (-21.8478, -13.9369, 7) (-20.25, -15.75, 7) (-18.4369, -17.3478, 7) (0, -17.5, 7) (18.4369, -17.3478, 7) (20.25, -15.75, 7) (21.8478, -13.9369, 7) (22, 0, 7) (21.8478, 13.9369, 7) (20.25, 15.75, 7) (18.4369, 17.3478, 7) (0, 17.5, 7) (-18.4369, 17.3478, 7) on bodies 1 in component "lid"
extrude "Extrude4" add sketch "Sketch3" along normal blind 5.5 from surface at 1.5 contours L0 L1 L2 L3 A0 L8 L9 L11 L18 L19 | L4 L5 L6 L7 A1 L12 L13 L15 L16 L17 bodies 1 in component "lid"
extrude "Extrude5" add sketch "Sketch3" along normal blind 3.5 from surface at 3.5 contours L2 A0 L9 L10 L11 A6 | L6 A1 L13 L14 L15 A7 bodies 1 in component "lid"
extrude "Extrude6" cut sketch "sma" along normal blind 4 from surface at 16 bodies 1 in component "lid"
extrude "Extrude7" cut sketch "panel" against normal blind 4 from surface at -16 bodies 1 in component "lid"
sketch "Sketch6" plane through (0, 0, 0) normal (0, 0, 1) x (1, 0, 0) in component "lid"
  line L0 (15.8, 8) -> (21.3, 8)
  line L1 (14.8, 9) -> (22.1, 9)
  line L2 (21.3, -4) -> (15.8, -4)
  line L3 (22.1, 9) -> (22.1, -5)
  line L4 (21.3, 8) -> (21.3, -4)
  line L5 (22.1, -5) -> (14.8, -5)
  line L6 (14.8, -5) -> (14.8, 9)
  line L7 (15.8, -4) -> (15.8, 8)
  dimension "d142" = 5.5
  dimension "d143" = 12
  dimension "d144" = 7.3
  dimension "d145" = 14
  constraint horizontal L0
  constraint vertical L4
  constraint horizontal L2
  constraint vertical L7
  constraint horizontal L1
  constraint vertical L3
  constraint horizontal L5
  constraint vertical L6
  measures "d142" distance of L0.start L0.end
  measures "d143" distance of L2.end L0.start
  measures "d144" distance of L1.start L1.end
  measures "d145" distance of L1.start L5.end
sketch "Sketch2 (2)" plane through (0, 0, 0) normal (0, 0, 1) x (1, 0, 0) in component "base"
  line L0 (-15.1, 19) -> (-8.6, 19)
  line L1 (-8.6, 19) -> (-8.6, 15.5)
  line L2 (-8.6, 15.5) -> (-15.1, 15.5)
  line L3 (-15.1, 15.5) -> (-15.1, 19)
  constraint horizontal L0
  constraint vertical L1
  constraint horizontal L2
  constraint vertical L3
extrude "Extrude4'" cut sketch "Sketch2 (2)" along normal blind 2 bodies 8 in component "base"
sketch "Sketch3 (2)" plane through (0, 0, 0) normal (0, 0, 1) x (1, 0, 0) in component "base"
  circle A0 centre (19, 14.4989) radius 1.25
  circle A1 centre (-19, -14.5102) radius 1.25
  dimension "d154" = 2.5
  dimension "d155" = 2.5
  measures "d154" diameter of A0
  measures "d155" diameter of A1
sketch "Sketch4" plane through (0, 0, 0) normal (0, 0, 1) x (1, 0, 0) in component "base"
  circle A0 through (21.5, 14.5, -2) (17.75, 16.6651, -2) (17.75, 12.3349, -2)
  circle A1 through (-16.5, -14.51, -2) (-20.25, -12.3449, -2) (-20.25, -16.6751, -2)
  dimension "d156" = 5
  dimension "d157" = 5
loft "Loft1" cut profiles "Sketch4", "Sketch3 (2)" section 1 contours A1 in plane through (0, 0, -2) normal (0, 0, 1) section 2 contours A1 bodies 8 in component "base"
loft "Loft2" cut profiles "Sketch4", "Sketch3 (2)" section 1 contours A0 in plane through (0, 0, -2) normal (0, 0, 1) section 2 contours A0 bodies 8 in component "base"
component "lid" placed x (1, 0, 0) y (0, 1, 0) z (0, 0, 1) at (0, 0, 0)
component "base" placed x (1, 0, 0) y (0, 1, 0) z (0, 0, 1) at (0, 0, 0)
equation "d4 = d3"
equation "d6 = d5"
equation "d8 = d7"
equation "d10 = d9"
equation "d12 = d11"
equation "d14 = d13"
equation "d16 = d15"
equation "d18 = d17"
equation "d40 = d39"
equation "d42 = d41"
equation "d44 = d43"
equation "d46 = d45"
equation "d55 = d54"
equation "d57 = d56"
equation "d59 = d58"
equation "d61 = d60"
equation "d69 = d68"
equation "d107 = d106"
equation "d109 = d108"
equation "d111 = d110"
equation "d113 = d112"
